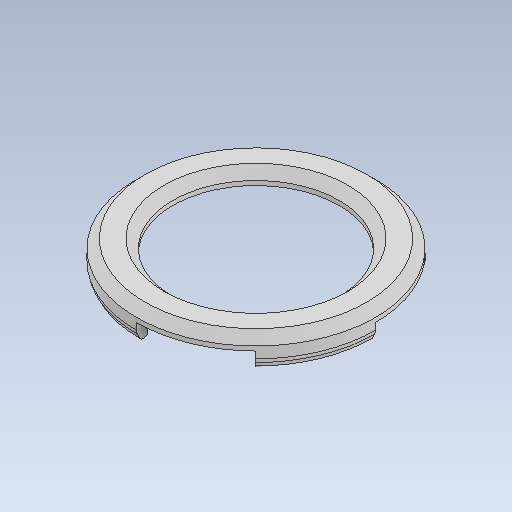
# Autodesk Inventor part: mirror_lock_v2
Saved by Autodesk Inventor 2020 (Build 240168000, 168)
## iProperties
Created: 2024-03-24
Part Number: mirror_lock_v2
Material: Типовые
Document SubType Name: Modeling
Designer: 4s
Density: 1 g/cm^3
Appearance: По умолчанию
Author: 4s
Autodesk Inventor part; units mm, degrees
ref_plane "YZ Plane" through (0, 0, 0) normal (1, 0, 0) x (0, 1, 0)
ref_plane "XZ Plane" through (0, 0, 0) normal (0, 1, 0) x (-1, 0, 0)
ref_plane "XY Plane" through (0, 0, 0) normal (0, 0, 1) x (1, 0, 0)
sketch "Эскиз1" plane through (0, 0, 0) normal (1, 0, 0) x (0, 1, 0)
  line L0 (0, 0) -> (10.522, 0) construction
  line L1 (0, 0) -> (0, -19) construction
  line L2 (0, 0) -> (0, -27.3) construction
  line L3 (0, -19) -> (3, -19)
  line L4 (3, -19) -> (3, -27.3)
  line L5 (3, -27.3) -> (0, -27.3)
  line L6 (0, -27.3) -> (0, -19)
  dimension "d0" = 19
  dimension "d1" = 27.3
  dimension "d2" = 3
  constraints: 14 end point, 2 horizontal, 2 parallel, 2 point on line, 1 perpendicular, 1 vertical
  measures "d0" distance of L0.start L1.end
  measures "d1" distance of L0.start L2.end
  measures "d2" distance of L4.end L5.end
revolve "Вращение1" add sketch "Эскиз1" angle 360 about axis through (0, 0, 0) along (0, 1, 0)
chamfer "Фаска1" distance 2 angle 45 1 edges at (0, 3, 19) measured on face at (2.1778, 3, -24.2689)
chamfer "Фаска2" distance 2 angle 45 1 edges at (0, 3, 27.3) measured on face at (3.853, 3, -24.7322)
sketch "Эскиз2" plane through (0, 0, 0) normal (1, 0, 0) x (0, 1, 0)
  line L0 (0, 0) -> (7.8289, 0) construction
  line L1 (0, 0) -> (0, -24.8) construction
  line L2 (0, 27.3) -> (0, -27.3) construction
  line L3 (0, -25.3) -> (-1.8, -25.3)
  line L4 (0, -27.3) -> (-1.5385, -27.3)
  line L5 (-2, -25.3) -> (-2, -26.7) construction
  line L6 (0, -25.3) -> (0, -27.3)
  line L7 (-2, 0.25) -> (-2, -25) construction
  line L8 (-2, -25) -> (-6, -25) construction
  arc A0 (-2.2, -25.1) -> (-3.4382, -26.5989) centre (-3, -25.7) ccw
  line L9 (-4, -25) -> (-4, 0) construction
  line L10 (-2, -24.7) -> (-4, -24.7) construction
  line L11 (-2, -25.3) -> (-2.0835, -25.3) construction
  arc A1 (-2, -25.7) -> (-2.0835, -25.3) centre (-3, -25.7) ccw construction
  arc A2 (-2.2, -25.1) -> (-1.8, -25.3) centre (-1.8, -24.8) ccw
  line L12 (-2.4149, -27.0978) -> (-3.4382, -26.5989)
  arc A3 (-3.4382, -26.5989) -> (-2, -25.7) centre (-3, -25.7) ccw construction
  arc A4 (-2.4149, -27.0978) -> (-1.5385, -27.3) centre (-1.5385, -25.3) ccw
  point P0 (-2.2859, -25)
  point P1 (-2, -27.3)
  dimension "d10" = 24.8
  dimension "d11" = 2
  dimension "d12" = 0.5
  dimension "d14" = 2
  dimension "d15" = 2
  dimension "d16" = 2
  dimension "d17" = 0.3
  dimension "d18" = 0.5
  dimension "d19" = 50
  dimension "d21" = 2
  dimension "d22" = 2
  constraints: 24 end point, 13 point on circle, 10 point on line, 10 tangent, 6 horizontal, 5 centre point, 3 vertical, 1 collinear, 1 midpoint
  measures "d10" distance of L0.start L1.end
  measures "d11" distance of L3.start L5.start
  measures "d12" distance from line of L1.end L3
  measures "d14" distance between parallel lines of L1 L7
  measures "d15" diameter of A0
  measures "d16" distance between parallel lines of L7 L9
  measures "d17" distance from line of point (-2.286, -25) L10
  measures "d18" radius of A2
  measures "d19" diameter of L8 L0
  measures "d21" distance of L2.end point (-2, -27.3)
  measures "d22" radius of A4
revolve "Вращение2" add sketch "Эскиз2" angle 45 about axis through (0, 0, 0) along (0, -1, 0)
pattern_circular "Круговой массив1" count 4 over 360 about axis through (0, 1.5, 0) along (0, -1, 0) of "Вращение2"
